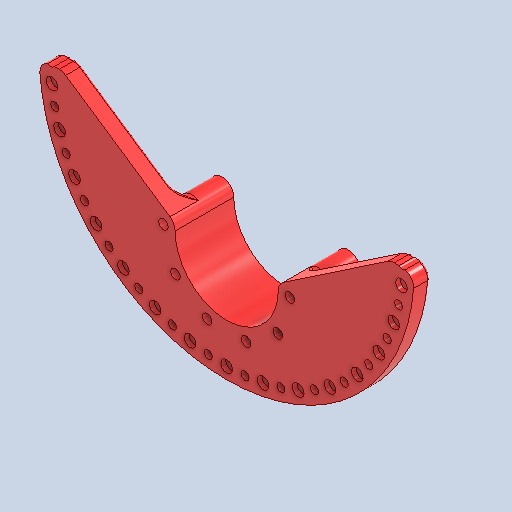
# Autodesk Inventor part: モーターマウント板固定部品2
Saved by Autodesk Inventor 2024 (Build 280153000, 153)
## iProperties
Created: 2023-05-30
Part Number: モーターマウント板固定部品2
Material: 一般
Document SubType Name: Modeling
Designer: yuta2
Density: 1 g/cm^3
Appearance: 淡い赤
Mass: 46.3632 g
Surface Area: 203.262 cm^2
Volume: 46.3632 cm^3
Author: yuta2
Autodesk Inventor part; units mm, degrees
ref_plane "YZ Plane" through (0, 0, 0) normal (1, 0, 0) x (0, 1, 0)
ref_plane "XZ Plane" through (0, 0, 0) normal (0, 1, 0) x (-1, 0, 0)
ref_plane "XY Plane" through (0, 0, 0) normal (0, 0, 1) x (1, 0, 0)
sketch "スケッチ1" plane through (0, 0, 0) normal (0, 0, 1) x (1, 0, 0)
  circle A0 centre (0, 0) radius 80
  circle A1 centre (0, 0) radius 70
  line L0 (-79.99375, -1) -> (79.99375, -1)
  line L1 (0, 0) -> (0, -80) construction
  arc A2 (-32, -36) -> (32, -36) centre (0, -36) ccw
  circle A3 centre (0, -36) radius 22
  arc A4 (-22, -36) -> (-32, -36) centre (-27, -36) ccw
  arc A5 (32, -36) -> (22, -36) centre (27, -36) ccw
  line L2 (-69.992857, -1) -> (-24.205912, -31.853547)
  line L3 (69.992857, -1) -> (24.205912, -31.853547)
  dimension "d0" = 160
  dimension "d1" = 10
  dimension "d2" = 1
  dimension "d3" = 64
  dimension "d4" = 44
  dimension "d5" = 36
  constraints: 15 point on circle, 8 end point, 6 centre point, 6 tangent, 3 point on line, 2 coincident, 2 horizontal alignment, 1 horizontal, 1 vertical
  measures "d0" diameter of A0
  measures "d1" radial gap between concentric circles of A0 A1
  measures "d2" distance from line of point (0, 0) L0
  measures "d3" diameter of A2
  measures "d4" diameter of A3
  measures "d5" distance of point (0, 0) A3.centre
extrude "押し出し1" add sketch "スケッチ1" along normal blind 7 contours L0 A1 A0 | L2 A4 A2 A5 L3 A1 | A4 A3 A5 A2 picked at (76.285294, -5.134296)
sketch "スケッチ2" plane through (0, 0, 7) normal (0, 0, 1) x (1, 0, 0)
  arc A0 (-79.99375, -1) -> (79.99375, -1) centre (0, 0) ccw
  line L0 (74.589142, -7.839635) -> (0, 0)
  line L1 (0, 0) -> (36.26862, 0)
  dimension "d8" = 6
  dimension "d9" = 75
  constraints: 4 end point, 1 horizontal
  measures "d8" angle of L0 L1
  measures "d9" distance of L0.start L0.end
hole "穴1" at (74.589142, -7.839635, 7) direction (0, 0, -1) diameter 5 depth 2
pattern_circular "円形状パターン1" count 30 over 360 about axis through (0, 0, 0) along (0, 0, 1) of "穴1"
sketch "スケッチ4" plane through (0, 0, 0) normal (0, 0, -1) x (-1, 0, 0)
  arc A0 (-22, -36) -> (22, -36) centre (0, -36) ccw
  circle A1 centre (0, -36) radius 32
  line L0 (-69.992857, -1) -> (-24.205912, -31.853547)
  line L1 (24.205912, -31.853547) -> (69.992857, -1)
  arc A2 (-30.8215, -27.395631) -> (30.8215, -27.395631) centre (0, -36) ccw
  line L2 (-69.992857, -1) -> (-24.205912, -31.853547)
  line L3 (-79.99375, -1) -> (-69.992857, -1)
  arc A3 (-79.99375, -1) -> (79.99375, -1) centre (0, 0) ccw
  line L4 (69.992857, -1) -> (79.99375, -1)
  line L5 (24.205912, -31.853547) -> (69.992857, -1)
  arc A4 (24.205912, -31.853547) -> (22, -36) centre (27, -36) ccw
  arc A5 (-22, -36) -> (22, -36) centre (0, -36) ccw
  arc A6 (-22, -36) -> (-24.205912, -31.853547) centre (-27, -36) ccw
  point P0 (22, -36)
  dimension "d20" = 64
  constraints: 4 point on circle, 2 centre point, 2 concentric, 2 point on line, 1 coincident
  measures "d20" diameter of A1
extrude "押し出し2" add sketch "スケッチ4" along normal blind 18 contours A0 A4 L1 A1 L0 A6 picked at (28.13802, -40.330295)
sketch "スケッチ5" plane through (0, 0, -18) normal (0, 0, -1) x (-1, 0, 0)
  arc A0 (-22, -36) -> (22, -36) centre (0, -36) ccw projected
  circle A1 centre (0, -36) radius 27
  point P0 (0, 0)
  point P1 (27, -36)
  dimension "d23" = 54
  constraints: 2 horizontal alignment, 1 coincident, 2 other
hole "穴2" at (-27, -36, -18) direction (0, 0, 1) diameter 4.1 end through all counterbore diameter 5.8 counterbore depth 4
pattern_circular "円形状パターン2" count 6 over 180 about axis through (0, -36, 0) along (0, 0, 1) of "穴2"
fillet "フィレット1" radius 5 2 edges at (30.8215, -27.3956, -9) (-30.8215, -27.3956, -9)
fillet "フィレット2" radius 5 3 edges at (0, -68, 0) (29.3484, -31.5857, 0) (-29.3484, -31.5857, 0)
fillet "フィレット3" radius 5 4 edges at (79.9937, -1, 3.5) (69.9929, -1, 3.5) (-79.9937, -1, 3.5) (-69.9929, -1, 3.5)
fillet "フィレット4" radius 1 15 edges at (0, -80, 0) (78.4338, -2.6088, 0) (73.1399, -1, 0) (70.0595, -1.2181, 0) (50.057, -14.4338, 0) (31.1044, -27.205, -0.0087) (27.1685, -29.8572, -1.8158) (-78.4338, -2.6088, 0) (-73.1399, -1, 0) (-70.0595, -1.2181, 0) (-50.057, -14.4338, 0) (-31.1044, -27.205, -0.0087) (-27.1685, -29.8572, -1.8158) (-24.206, -31.8535, -4.9999) (-24.2059, -31.8535, -4.9999)
sketch "スケッチ6" plane through (0, 0, 0) normal (0, 0, -1) x (-1, 0, 0)
  arc A0 (-22, -36) -> (22, -36) centre (0, -36) ccw
  line L0 (0, -36) -> (0, 0)
  line L1 (0, 0) -> (8.362277, -79.561752)
  arc A1 (-79.743589, -6.4) -> (79.743589, -6.4) centre (0, 0) ccw
  circle A2 centre (0, 0) radius 75
  point P0 (7.839635, -74.589142)
  dimension "d39" = 150
  dimension "d38" = 6
  constraints: 4 end point, 1 coincident, 1 point on circle, 1 point on line, 1 vertical, 3 other
  measures "d38" angle of L1 L0
hole "穴3" at (-7.839635, -74.589142, 0) direction (0, 0, 1) diameter 3.5 end through all
pattern_circular "円形状パターン3" count 30 over 360 about axis through (0, 0, 1) along (0, 0, 1) of "穴3"
equation "\"d9\" = 0.5 * D"
equation "\"d39\" = D"
equation "\"D\" = 150"
